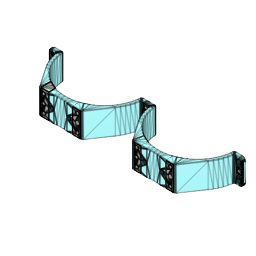
double_berceau (Autodesk Fusion 360 design; units mm, degrees)
Autodesk Fusion 360 part; units mm, degrees
other "Fonction de maillage de base1"
other "CopierCollerMaillages1"
other "Modifier1"
sketch "Esquisse1" plane through (0, 0, 0) normal (0, 1, 0) x (1, 0, 0)
  line L0 (362.8776, -300) -> (460, -300)
  line L1 (460, -300) -> (460, -7.248)
  line L2 (460, -7.248) -> (362.8776, -7.248)
  line L3 (362.8776, -7.248) -> (362.8776, -300)
  line L4 (740, -290) -> (836.9455, -290)
  line L5 (836.9455, -290) -> (836.9455, -5.3756)
  line L6 (836.9455, -5.3756) -> (740, -5.3756)
  line L7 (740, -5.3756) -> (740, -290)
  line L8 (1467.8104, -290) -> (1550, -290)
  line L9 (1550, -290) -> (1550, -8.5838)
  line L10 (1550, -8.5838) -> (1467.8104, -8.5838)
  line L11 (1467.8104, -8.5838) -> (1467.8104, -290)
  line L12 (1846.0065, -290.6538) -> (1934.374, -290.6538)
  line L13 (1934.374, -290.6538) -> (1934.374, -7.03)
  line L14 (1934.374, -7.03) -> (1846.0065, -7.03)
  line L15 (1846.0065, -7.03) -> (1846.0065, -290.6538)
  constraint horizontal L0
  constraint vertical L1
  constraint horizontal L2
  constraint vertical L3
  constraint horizontal L4
  constraint vertical L5
  constraint horizontal L6
  constraint vertical L7
  constraint horizontal L8
  constraint vertical L9
  constraint horizontal L10
  constraint vertical L11
  constraint horizontal L12
  constraint vertical L13
  constraint horizontal L14
  constraint vertical L15
extrude "Extrusion1" add sketch "Esquisse1" along normal blind 200 makes body 1 at (740, 66.6667, 100.2504) makes body 2 at (1467.8104, 66.6667, 102.3892) makes body 3 at (362.8776, 66.6667, 104.832) makes body 4 at (1846.0065, 66.6667, 101.5712)
sketch "Esquisse3" plane through (0, 0, 0) normal (0, 0, 1) x (1, 0, 0)
  circle A0 centre (597.2253, 517.7779) radius 458.2627
  circle A1 centre (1697.1609, 520.5175) radius 460.8616
extrude "Extrusion2" cut sketch "Esquisse3" along normal mid plane 5900 bodies 1 2 3 4
ref_plane "Plan de construction1" through (0, 500, 0) normal (0, 1, 0) x (0, 0, 1)
sketch "Esquisse4" plane through (0, 500, 0) normal (0, 1, 0) x (1, 0, 0)
  line L0 (10.3484, -195.5854) -> (80, -195.5854)
  line L1 (80, -195.5854) -> (80, -110)
  line L2 (80, -110) -> (10.3484, -110)
  line L3 (10.3484, -110) -> (10.3484, -195.5854)
  line L4 (1118.7094, -283.817) -> (1180, -283.817)
  line L5 (1180, -283.817) -> (1180, -220)
  line L6 (1180, -220) -> (1118.7094, -220)
  line L7 (1118.7094, -220) -> (1118.7094, -283.817)
  line L8 (1122.2231, -82.7582) -> (1180, -82.7582)
  line L9 (1180, -82.7582) -> (1180, -20)
  line L10 (1180, -20) -> (1122.2231, -20)
  line L11 (1122.2231, -20) -> (1122.2231, -82.7582)
  line L12 (2220, -180) -> (2280, -180)
  line L13 (2280, -180) -> (2280, -120)
  line L14 (2280, -120) -> (2220, -120)
  line L15 (2220, -120) -> (2220, -180)
  constraint horizontal L0
  constraint vertical L1
  constraint horizontal L2
  constraint vertical L3
  constraint horizontal L4
  constraint vertical L5
  constraint horizontal L6
  constraint vertical L7
  constraint horizontal L8
  constraint vertical L9
  constraint horizontal L10
  constraint vertical L11
  constraint horizontal L12
  constraint vertical L13
  constraint horizontal L14
  constraint vertical L15
extrude "Extrusion3" add sketch "Esquisse4" against normal blind 40 separate body makes body 5 at (1139.1396, 500, 241.2723) makes body 6 at (1141.4821, 500, 40.9194) makes body 7 at (56.7828, 500, 138.5285) makes body 8 at (2240, 500, 140)
sketch "Esquisse5" plane through (0, 500, 0) normal (0, 1, 0) x (1, 0, 0)
scale "Echelle1" factor 1 about (596.8149, 250.025, 150.0002) bodies 3 1 6 5 7 2 4 8
other "Echelle1'"
scale "Echelle2" factor 0.1 about (10.3484, 500, 195.5854) bodies 7 1 3 5 6 2 4 8
other "Echelle2'"
sketch "Esquisse6" plane through (0, 500, 0) normal (0, 1, 0) x (1, 0, 0)
